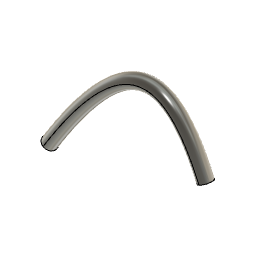
Final assembly_1001 (Autodesk Fusion 360 archive; units mm, degrees)
design "Blow Pipe_1001"
Autodesk Fusion 360 part; units mm, degrees
sketch "Sketch1" plane through (0, 0, 0) normal (0, 1, 0) x (1, 0, 0)
  spline S0 degree 5 poles (0, 0) (-0.9955, -2.3111) (-3.0243, -6.6799) (-6.1809, -12.4734) (-10.6201, -18.6535) (-16.5766, -23.6475) (-22.9681, -25.7259) (-29.8145, -24.7556) (-37.1022, -20.8271) (-44.7943, -14.1881) (-52.8502, -5.111) (-59.5578, 3.9127) (-64.7263, 11.6033) (-68.2321, 17.1339) (-70, 20) knots 0 0 0 0 0 0 0.1 0.2 0.3 0.4 0.5 0.6 0.7 0.8 0.9 1 1 1 1 1 1
  point P0 (-25, -25)
  constraint coincident S0.start origin
pipe "Pipe1" add diameter 6 wall 1 path "Sketch1" along S0

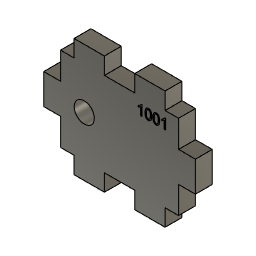
design "Housing block blowtube side version 2"
Autodesk Fusion 360 part; units mm, degrees
sketch "Sketch1" plane through (0, 0, 0) normal (0, 1, 0) x (1, 0, 0)
  line L0 (9, -55) -> (9, -50)
  line L1 (9, -50) -> (5, -50)
  line L2 (36, -55) -> (36, -50)
  line L3 (36, -50) -> (40, -50)
  line L4 (9, -55) -> (18, -55)
  line L5 (18, -55) -> (18, -50)
  line L6 (18, -50) -> (27, -50)
  line L7 (27, -50) -> (27, -55)
  line L8 (9, -55) -> (18, -55)
  line L9 (27, -55) -> (36, -55)
  line L10 (4, -42) -> (0, -42)
  line L11 (41, -42) -> (45, -42)
  line L12 (0, -42) -> (0, -37.5)
  line L13 (45, -42) -> (45, -37.5)
  line L14 (0, -37.5) -> (45, -37.5) construction
  line L15 (4, -42) -> (5, -42)
  line L16 (5, -42) -> (5, -50)
  line L17 (41, -42) -> (40, -42)
  line L18 (40, -42) -> (40, -50)
  line L19 (9, -20) -> (18, -20)
  line L20 (5, -33) -> (5, -25)
  line L21 (41, -33) -> (40, -33)
  line L22 (9, -25) -> (5, -25)
  line L23 (36, -20) -> (36, -25)
  line L24 (40, -33) -> (40, -25)
  line L25 (27, -25) -> (27, -20)
  line L26 (4, -33) -> (5, -33)
  line L27 (18, -25) -> (27, -25)
  line L28 (18, -20) -> (18, -25)
  line L29 (27, -20) -> (36, -20)
  line L30 (9, -20) -> (9, -25)
  line L31 (36, -25) -> (40, -25)
  line L32 (9, -20) -> (18, -20)
  line L33 (41, -33) -> (45, -33)
  line L34 (4, -33) -> (0, -33)
  line L35 (45, -33) -> (45, -37.5)
  line L36 (0, -33) -> (0, -37.5)
  dimension "d3" = 4.5
  dimension "d4" = 4.5
  constraint horizontal L8
  constraint vertical L0
  constraint horizontal L1
  constraint vertical L2
  constraint horizontal L3
  constraint perpendicular L4 L5
  constraint perpendicular L5 L6
  constraint coincident L7.end L8
  constraint perpendicular L7 L8
  constraint collinear L8 L9
  constraint perpendicular L10 L12
  constraint perpendicular L11 L13
  constraint perpendicular L13 L14
  constraint perpendicular L1 L16
  constraint perpendicular L3 L18
  constraint symmetric L0.start L14 L19.start
  constraint symmetric L0.end L14 L22.start
  constraint symmetric L2.start L14 L23.start
  constraint symmetric L2.end L14 L23.end
  constraint symmetric L4.end L14 L19.end
  constraint symmetric L5.end L14 L27.start
  constraint symmetric L6.end L14 L25.start
  constraint symmetric L7.end L14 L25.end
  constraint symmetric L10.start L14 L26.start
  constraint symmetric L10.end L14 L34.end
  constraint symmetric L11.start L14 L21.start
  constraint symmetric L11.end L14 L33.end
  constraint symmetric L12.end L14 L36.end
  constraint symmetric L13.end L14 L35.end
  constraint symmetric L14 L15.end L20.start
  constraint symmetric L14 L1.end L20.end
  constraint symmetric L14 L17.end L21.end
  constraint symmetric L14 L3.end L24.end
  measures "d3" distance of L10.end L12.end
  measures "d4" distance of L11.end L13.end
extrude "Extrude1" add sketch "Sketch1" along normal blind 5
sketch "Sketch2" plane through (0, 0, 0) normal (0, -1, 0) x (1, 0, 0)
  line L0 (0, 33) -> (5, 33)
  line L1 (5, 33) -> (5, 25)
  line L2 (5, 25) -> (9, 25)
  line L3 (9, 25) -> (9, 20)
  line L4 (9, 20) -> (18, 20)
  line L5 (18, 20) -> (18, 25)
  line L6 (18, 25) -> (27, 25)
  line L7 (27, 25) -> (27, 20)
  line L8 (27, 20) -> (36, 20)
  line L9 (36, 20) -> (36, 25)
  line L10 (36, 25) -> (40, 25)
  line L11 (40, 25) -> (40, 33)
  line L12 (40, 33) -> (45, 33)
  line L13 (45, 33) -> (45, 42)
  line L14 (45, 42) -> (40, 42)
  line L15 (40, 42) -> (40, 50)
  line L16 (40, 50) -> (36, 50)
  line L17 (36, 50) -> (36, 55)
  line L18 (36, 55) -> (27, 55)
  line L19 (27, 55) -> (27, 50)
  line L20 (27, 50) -> (18, 50)
  line L21 (18, 50) -> (18, 55)
  line L22 (18, 55) -> (9, 55)
  line L23 (9, 55) -> (9, 50)
  line L24 (9, 50) -> (5, 50)
  line L25 (5, 50) -> (5, 42)
  line L26 (5, 42) -> (0, 42)
  line L27 (0, 42) -> (0, 33)
  circle A0 centre (12.027, 37.5) radius 3
  dimension "d7" = 6
  measures "d7" diameter of A0
extrude "Extrude2" cut sketch "Sketch2" against normal blind 5 contours A0
sketch "Sketch3" plane through (0, 0, 0) normal (0, -1, 0) x (1, 0, 0)
  circle A0 centre (12.027, 37.5) radius 3
  line L0 (0, 33) -> (5, 33)
  line L1 (5, 33) -> (5, 25)
  line L2 (5, 25) -> (9, 25)
  line L3 (9, 25) -> (9, 20)
  line L4 (9, 20) -> (18, 20)
  line L5 (18, 20) -> (18, 25)
  line L6 (18, 25) -> (27, 25)
  line L7 (27, 25) -> (27, 20)
  line L8 (27, 20) -> (36, 20)
  line L9 (36, 20) -> (36, 25)
  line L10 (36, 25) -> (40, 25)
  line L11 (40, 25) -> (40, 33)
  line L12 (40, 33) -> (45, 33)
  line L13 (45, 33) -> (45, 42)
  line L14 (45, 42) -> (40, 42)
  line L15 (40, 42) -> (40, 50)
  line L16 (40, 50) -> (36, 50)
  line L17 (36, 50) -> (36, 55)
  line L18 (36, 55) -> (27, 55)
  line L19 (27, 55) -> (27, 50)
  line L20 (27, 50) -> (18, 50)
  line L21 (18, 50) -> (18, 55)
  line L22 (18, 55) -> (9, 55)
  line L23 (9, 55) -> (9, 50)
  line L24 (9, 50) -> (5, 50)
  line L25 (5, 50) -> (5, 42)
  line L26 (5, 42) -> (0, 42)
  line L27 (0, 42) -> (0, 33)
  line L28 (27.9971, 44.0065) -> (37, 44) construction
  line L29 (37, 44) -> (37.0029, 47.9935) construction
  line L30 (37.0029, 47.9935) -> (28, 48) construction
  line L31 (28, 48) -> (27.9971, 44.0065) construction
  dimension "d10" = 3
  text T0 "1001" font "Arial" height 3 align left top in box 9.0029 x 3.9935 at (27.9971, 44.0065) x (1, -0.000717) y (0.000717, 1) spacing 1 kerned
emboss "Emboss1" depth -0.1 profiles "Sketch3" section 1 text T0 onto face at (31.3333, 0, 36)

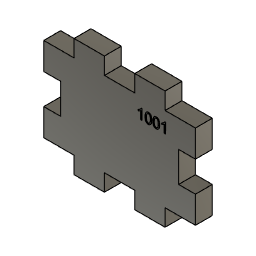
design "Housing block top and bottom version 2"
Autodesk Fusion 360 part; units mm, degrees
sketch "Sketch1" plane through (0, 0, 0) normal (0, 1, 0) x (1, 0, 0)
  line L0 (45, -22) -> (45, -30)
  line L1 (0, -30) -> (9, -30)
  line L2 (9, -30) -> (9, -35)
  line L3 (9, -35) -> (18, -35)
  line L4 (18, -35) -> (18, -30)
  line L5 (18, -30) -> (27, -30)
  line L6 (27, -30) -> (27, -35)
  line L7 (36, -35) -> (27, -35)
  line L8 (18, -35) -> (9, -35)
  line L9 (36, -35) -> (36, -30)
  line L10 (36, -30) -> (45, -30)
  line L11 (0, -30) -> (0, -22)
  line L12 (5, -22) -> (5, -17.5)
  line L13 (45, -30) -> (45, -22)
  line L14 (40, -22) -> (40, -17.5)
  line L15 (40, -22) -> (45, -22)
  line L16 (5, -17.5) -> (40, -17.5) construction
  line L17 (18, 0) -> (9, 0)
  line L18 (27, -5) -> (27, 0)
  line L19 (36, -5) -> (45, -5)
  line L20 (36, 0) -> (27, 0)
  line L21 (18, 0) -> (18, -5)
  line L22 (9, 0) -> (18, 0)
  line L23 (40, -13) -> (45, -13)
  line L24 (0, -5) -> (0, -13)
  line L25 (18, -5) -> (27, -5)
  line L26 (0, -5) -> (9, -5)
  line L27 (40, -13) -> (40, -17.5)
  line L28 (36, 0) -> (36, -5)
  line L29 (5, -13) -> (5, -17.5)
  line L30 (9, -5) -> (9, 0)
  line L31 (45, -5) -> (45, -13)
  line L32 (0, -22) -> (5, -22)
  line L33 (5, -13) -> (0, -13)
  dimension "d3" = 4.5
  dimension "d4" = 4.5
  constraint vertical L0
  constraint horizontal L7
  constraint coincident L2.end L7
  constraint perpendicular L2 L7
  constraint coincident L3.end L7
  constraint perpendicular L3 L4
  constraint perpendicular L4 L5
  constraint perpendicular L6 L7
  constraint collinear L7 L8
  constraint perpendicular L7 L9
  constraint perpendicular L0 L10
  constraint perpendicular L1 L12
  constraint perpendicular L10 L14
  constraint perpendicular L13 L15
  constraint perpendicular L12 L16
  constraint symmetric L1.start L16 L24.start
  constraint symmetric L1.end L16 L26.end
  constraint symmetric L2.end L16 L17.end
  constraint symmetric L3.end L16 L17.start
  constraint symmetric L4.end L16 L21.end
  constraint symmetric L5.end L16 L18.start
  constraint symmetric L6.end L16 L18.end
  constraint symmetric L7.start L16 L20.start
  constraint symmetric L9.end L16 L19.start
  constraint symmetric L0.end L16 L19.end
  constraint symmetric L11.end L16 L24.end
  constraint symmetric L12.start L16 L29.start
  constraint symmetric L12.end L16 L29.end
  constraint symmetric L0.start L16 L23.end
  constraint symmetric L14.start L16 L23.start
  constraint symmetric L14.end L16 L27.end
  constraint perpendicular L11 L32
  measures "d3" distance of L12.start L12.end
  measures "d4" distance of L14.start L14.end
extrude "Extrude1" add sketch "Sketch1" along normal blind 5
sketch "Sketch2" plane through (0, 0, 0) normal (0, -1, 0) x (1, 0, 0)
  line L0 (9, 30) -> (0, 30)
  line L1 (0, 30) -> (0, 22)
  line L2 (0, 22) -> (5, 22)
  line L3 (5, 22) -> (5, 13)
  line L4 (5, 13) -> (0, 13)
  line L5 (0, 13) -> (0, 5)
  line L6 (0, 5) -> (9, 5)
  line L7 (9, 5) -> (9, 0)
  line L8 (9, 0) -> (18, 0)
  line L9 (18, 0) -> (18, 5)
  line L10 (18, 5) -> (27, 5)
  line L11 (27, 5) -> (27, 0)
  line L12 (27, 0) -> (36, 0)
  line L13 (36, 0) -> (36, 5)
  line L14 (36, 5) -> (45, 5)
  line L15 (45, 5) -> (45, 13)
  line L16 (45, 13) -> (40, 13)
  line L17 (40, 13) -> (40, 22)
  line L18 (40, 22) -> (45, 22)
  line L19 (45, 22) -> (45, 30)
  line L20 (45, 30) -> (36, 30)
  line L21 (36, 30) -> (36, 35)
  line L22 (36, 35) -> (27, 35)
  line L23 (27, 35) -> (27, 30)
  line L24 (27, 30) -> (18, 30)
  line L25 (18, 30) -> (18, 35)
  line L26 (18, 35) -> (9, 35)
  line L27 (9, 35) -> (9, 30)
  line L28 (27.994, 23.0136) -> (37, 23) construction
  line L29 (37, 23) -> (37.006, 26.9864) construction
  line L30 (37.006, 26.9864) -> (28, 27) construction
  line L31 (28, 27) -> (27.994, 23.0136) construction
  dimension "d7" = 3
  text T0 "1001" font "Arial" height 3 align left top in box 9.006 x 3.9864 at (27.994, 23.0136) x (0.999999, -0.001514) y (0.001514, 0.999999) spacing 1 kerned
emboss "Emboss1" depth -0.1 profiles "Sketch2" section 1 text T0 onto face at (13.6667, 0, 17.5)

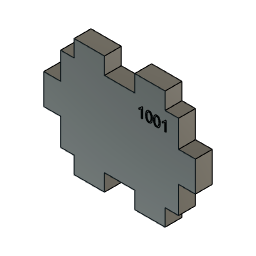
design "Housing block other side version 2"
Autodesk Fusion 360 part; units mm, degrees
sketch "Sketch1" plane through (0, 0, 0) normal (0, 1, 0) x (1, 0, 0)
  line L0 (9, -55) -> (9, -50)
  line L1 (9, -50) -> (5, -50)
  line L2 (36, -55) -> (36, -50)
  line L3 (36, -50) -> (40, -50)
  line L4 (9, -55) -> (18, -55)
  line L5 (18, -55) -> (18, -50)
  line L6 (18, -50) -> (27, -50)
  line L7 (27, -50) -> (27, -55)
  line L8 (9, -55) -> (18, -55)
  line L9 (27, -55) -> (36, -55)
  line L10 (4, -42) -> (0, -42)
  line L11 (41, -42) -> (45, -42)
  line L12 (0, -42) -> (0, -37.5)
  line L13 (45, -42) -> (45, -37.5)
  line L14 (0, -37.5) -> (45, -37.5) construction
  line L15 (4, -42) -> (5, -42)
  line L16 (5, -42) -> (5, -50)
  line L17 (41, -42) -> (40, -42)
  line L18 (40, -42) -> (40, -50)
  line L19 (9, -20) -> (18, -20)
  line L20 (5, -33) -> (5, -25)
  line L21 (41, -33) -> (40, -33)
  line L22 (9, -25) -> (5, -25)
  line L23 (36, -20) -> (36, -25)
  line L24 (40, -33) -> (40, -25)
  line L25 (27, -25) -> (27, -20)
  line L26 (4, -33) -> (5, -33)
  line L27 (18, -25) -> (27, -25)
  line L28 (18, -20) -> (18, -25)
  line L29 (27, -20) -> (36, -20)
  line L30 (9, -20) -> (9, -25)
  line L31 (36, -25) -> (40, -25)
  line L32 (9, -20) -> (18, -20)
  line L33 (41, -33) -> (45, -33)
  line L34 (4, -33) -> (0, -33)
  line L35 (45, -33) -> (45, -37.5)
  line L36 (0, -33) -> (0, -37.5)
  dimension "d3" = 4.5
  dimension "d4" = 4.5
  constraint horizontal L8
  constraint vertical L0
  constraint horizontal L1
  constraint vertical L2
  constraint horizontal L3
  constraint perpendicular L4 L5
  constraint perpendicular L5 L6
  constraint coincident L7.end L8
  constraint perpendicular L7 L8
  constraint collinear L8 L9
  constraint perpendicular L10 L12
  constraint perpendicular L11 L13
  constraint perpendicular L13 L14
  constraint perpendicular L1 L16
  constraint perpendicular L3 L18
  constraint symmetric L0.start L14 L19.start
  constraint symmetric L0.end L14 L22.start
  constraint symmetric L2.start L14 L23.start
  constraint symmetric L2.end L14 L23.end
  constraint symmetric L4.end L14 L19.end
  constraint symmetric L5.end L14 L27.start
  constraint symmetric L6.end L14 L25.start
  constraint symmetric L7.end L14 L25.end
  constraint symmetric L10.start L14 L26.start
  constraint symmetric L10.end L14 L34.end
  constraint symmetric L11.start L14 L21.start
  constraint symmetric L11.end L14 L33.end
  constraint symmetric L12.end L14 L36.end
  constraint symmetric L13.end L14 L35.end
  constraint symmetric L14 L15.end L20.start
  constraint symmetric L14 L1.end L20.end
  constraint symmetric L14 L17.end L21.end
  constraint symmetric L14 L3.end L24.end
  measures "d3" distance of L10.end L12.end
  measures "d4" distance of L11.end L13.end
extrude "Extrude1" add sketch "Sketch1" along normal blind 5
sketch "Sketch2" plane through (0, 0, 0) normal (0, -1, 0) x (1, 0, 0)
  line L0 (0, 33) -> (5, 33)
  line L1 (5, 33) -> (5, 25)
  line L2 (5, 25) -> (9, 25)
  line L3 (9, 25) -> (9, 20)
  line L4 (9, 20) -> (18, 20)
  line L5 (18, 20) -> (18, 25)
  line L6 (18, 25) -> (27, 25)
  line L7 (27, 25) -> (27, 20)
  line L8 (27, 20) -> (36, 20)
  line L9 (36, 20) -> (36, 25)
  line L10 (36, 25) -> (40, 25)
  line L11 (40, 25) -> (40, 33)
  line L12 (40, 33) -> (45, 33)
  line L13 (45, 33) -> (45, 42)
  line L14 (45, 42) -> (40, 42)
  line L15 (40, 42) -> (40, 50)
  line L16 (40, 50) -> (36, 50)
  line L17 (36, 50) -> (36, 55)
  line L18 (36, 55) -> (27, 55)
  line L19 (27, 55) -> (27, 50)
  line L20 (27, 50) -> (18, 50)
  line L21 (18, 50) -> (18, 55)
  line L22 (18, 55) -> (9, 55)
  line L23 (9, 55) -> (9, 50)
  line L24 (9, 50) -> (5, 50)
  line L25 (5, 50) -> (5, 42)
  line L26 (5, 42) -> (0, 42)
  line L27 (0, 42) -> (0, 33)
sketch "Sketch3" plane through (0, 0, 0) normal (0, -1, 0) x (1, 0, 0)
  line L0 (28.1867, 44.4859) -> (37.0015, 44.4949) construction
  line L1 (37.0015, 44.4949) -> (36.9985, 47.5051) construction
  line L2 (36.9985, 47.5051) -> (28.1836, 47.4961) construction
  line L3 (28.1836, 47.4961) -> (28.1867, 44.4859) construction
  dimension "d8" = 3
  text T0 "1001" font "Arial" height 3 align left top in box 8.8149 x 3.0103 at (28.1867, 44.4859) x (0.999999, 0.00102) y (-0.00102, 0.999999) spacing 1 kerned
emboss "Emboss1" depth -0.1 profiles "Sketch3" section 1 text T0 onto face at (13.6667, 0, 36)

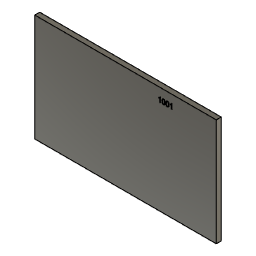
design "Base Plate"
Autodesk Fusion 360 part; units mm, degrees
sketch "Sketch1" plane through (0, 0, 0) normal (0, 1, 0) x (1, 0, 0)
  line L0 (-40, -25) -> (70, -25)
  line L1 (70, -25) -> (70, -90)
  line L2 (70, -90) -> (-40, -90)
  line L3 (-40, -90) -> (-40, -25)
  dimension "d1" = 110
  dimension "d2" = 65
  constraint horizontal L0
  constraint vertical L1
  constraint horizontal L2
  constraint vertical L3
  measures "d1" distance of L0.start L0.end
  measures "d2" distance of L0.start L2.end
extrude "Extrude1" add sketch "Sketch1" along normal blind 3
sketch "Sketch2" plane through (0, 0, 0) normal (0, -1, 0) x (1, 0, 0)
  line L0 (70, 90) -> (-40, 90)
  line L1 (-40, 90) -> (-40, 25)
  line L2 (-40, 25) -> (70, 25)
  line L3 (70, 25) -> (70, 90)
  line L4 (35, 75.5912) -> (62.1454, 75.5912) construction
  line L5 (62.1454, 75.5912) -> (62.1454, 85) construction
  line L6 (62.1454, 85) -> (35, 85) construction
  line L7 (35, 85) -> (35, 75.5912) construction
  dimension "d5" = 3
  text T0 "1001" font "Arial" height 3 align left top in box 27.1454 x 9.4088 at (35, 75.5912) x (1, 0) y (0, 1) spacing 1 kerned
emboss "Emboss1" depth -0.5 profiles "Sketch2" section 1 text T0 onto face at (-3.3333, 0, 46.6667)

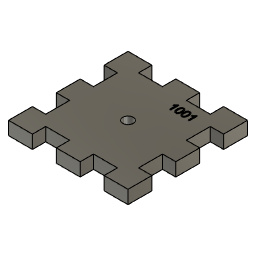
design "Housing_back"
Autodesk Fusion 360 part; units mm, degrees
sketch "Sketch1" plane through (0, 0, 0) normal (0, 0, 1) x (1, 0, 0)
  line L0 (0, 0) -> (9, 0)
  line L1 (9, 0) -> (9, -5)
  line L2 (9, -5) -> (18, -5)
  line L3 (18, -5) -> (18, 0)
  line L4 (18, 0) -> (27, 0)
  line L5 (27, 0) -> (27, -5)
  line L6 (27, -5) -> (36, -5)
  line L7 (36, -5) -> (36, 0)
  line L8 (36, 0) -> (45, 0)
  line L9 (45, 0) -> (45, -9)
  line L10 (45, -9) -> (40, -9)
  line L11 (40, -9) -> (40, -18)
  line L12 (40, -18) -> (45, -18)
  line L13 (45, -18) -> (45, -27)
  line L14 (45, -27) -> (40, -27)
  line L15 (40, -27) -> (40, -36)
  line L16 (40, -36) -> (45, -36)
  line L17 (45, -36) -> (45, -45)
  line L18 (50, 0) -> (50, -22.5) construction
  line L19 (50, -22.5) -> (-20, -22.5) construction
  line L20 (0, -45) -> (9, -45)
  line L21 (9, -45) -> (9, -40)
  line L22 (9, -40) -> (18, -40)
  line L23 (18, -40) -> (18, -45)
  line L24 (18, -45) -> (27, -45)
  line L25 (27, -45) -> (27, -40)
  line L26 (27, -40) -> (36, -40)
  line L27 (36, -40) -> (36, -45)
  line L28 (36, -45) -> (45, -45)
  line L29 (50, 0) -> (27.5, 0) construction
  line L30 (45, 10) -> (22.5, 10) construction
  line L31 (22.5, 10) -> (22.5, -55) construction
  line L32 (0, 0) -> (0, -9)
  line L33 (0, -9) -> (5, -9)
  line L34 (5, -9) -> (5, -18)
  line L35 (5, -18) -> (0, -18)
  line L36 (0, -18) -> (0, -27)
  line L37 (0, -27) -> (5, -27)
  line L38 (5, -27) -> (5, -36)
  line L39 (5, -36) -> (0, -36)
  line L40 (0, -36) -> (0, -45)
  dimension "d1" = 9
  dimension "d2" = 5
  dimension "d3" = 9
  dimension "d4" = 5
  dimension "d5" = 9
  dimension "d6" = 5
  dimension "d7" = 9
  dimension "d8" = 5
  dimension "d9" = 9
  dimension "d10" = 9
  dimension "d11" = 5
  dimension "d12" = 9
  dimension "d13" = 9
  dimension "d14" = 5
  dimension "d15" = 9
  dimension "d16" = 9
  dimension "d17" = 22.5
  dimension "d18" = 22.5
  dimension "d19" = 22.5
  constraint coincident L0.start L32.start
  constraint horizontal L0
  constraint perpendicular L0 L1
  constraint perpendicular L1 L2
  constraint perpendicular L2 L3
  constraint perpendicular L3 L4
  constraint perpendicular L4 L5
  constraint perpendicular L5 L6
  constraint perpendicular L6 L7
  constraint perpendicular L7 L8
  constraint perpendicular L8 L9
  constraint perpendicular L9 L10
  constraint perpendicular L10 L11
  constraint perpendicular L11 L12
  constraint perpendicular L12 L13
  constraint perpendicular L13 L14
  constraint perpendicular L14 L15
  constraint perpendicular L15 L16
  constraint perpendicular L16 L17
  constraint vertical L18
  constraint perpendicular L18 L19
  constraint symmetric L0.start L19 L20.start
  constraint symmetric L0.end L19 L20.end
  constraint symmetric L1.end L19 L21.end
  constraint symmetric L2.end L19 L22.end
  constraint symmetric L3.end L19 L23.end
  constraint symmetric L4.end L19 L24.end
  constraint symmetric L5.end L19 L25.end
  constraint symmetric L6.end L19 L26.end
  constraint symmetric L7.end L19 L27.end
  constraint symmetric L8.end L19 L17.end
  constraint perpendicular L9 L29
  constraint perpendicular L9 L30
  constraint perpendicular L24 L31
  constraint symmetric L8.end L31 L0.start
  constraint symmetric L9.end L31 L32.end
  constraint symmetric L10.end L31 L33.end
  constraint symmetric L11.end L31 L34.end
  constraint symmetric L12.end L31 L35.end
  constraint symmetric L13.end L31 L36.end
  constraint symmetric L14.end L31 L37.end
  constraint symmetric L15.end L31 L38.end
  constraint symmetric L16.end L31 L39.end
  constraint symmetric L17.end L31 L20.start
  measures "d1" distance of L0.start L0.end
  measures "d2" distance of L0.end L1.end
  measures "d3" distance of L1.end L2.end
  measures "d4" distance of L2.end L3.end
  measures "d5" distance of L3.end L4.end
  measures "d6" distance of L4.end L5.end
  measures "d7" distance of L5.end L6.end
  measures "d8" distance of L6.end L7.end
  measures "d9" distance of L7.end L8.end
  measures "d10" distance of L8.end L9.end
  measures "d11" distance of L9.end L10.end
  measures "d12" distance of L10.end L11.end
  measures "d13" distance of L12.end L13.end
  measures "d14" distance of L13.end L14.end
  measures "d15" distance of L14.end L15.end
  measures "d16" distance of L16.end L17.end
  measures "d17" distance of L18.start L18.end
  measures "d18" distance of L18.start L29.end
  measures "d19" distance of L30.start L30.end
extrude "Extrude1" add sketch "Sketch1" along normal blind 5
sketch "Sketch2" plane through (0, 0, 5) normal (0, 0, 1) x (-1, 0, 0)
  line L0 (0, 0) -> (0, 9)
  line L1 (0, 9) -> (-5, 9)
  line L2 (-5, 9) -> (-5, 18)
  line L3 (-5, 18) -> (0, 18)
  line L4 (0, 18) -> (0, 27)
  line L5 (0, 27) -> (-5, 27)
  line L6 (-5, 27) -> (-5, 36)
  line L7 (-5, 36) -> (0, 36)
  line L8 (0, 36) -> (0, 45)
  line L9 (0, 45) -> (-9, 45)
  line L10 (-9, 45) -> (-9, 40)
  line L11 (-9, 40) -> (-18, 40)
  line L12 (-18, 40) -> (-18, 45)
  line L13 (-18, 45) -> (-27, 45)
  line L14 (-27, 45) -> (-27, 40)
  line L15 (-27, 40) -> (-36, 40)
  line L16 (-36, 40) -> (-36, 45)
  line L17 (-36, 45) -> (-45, 45)
  line L18 (-45, 45) -> (-45, 36)
  line L19 (-45, 36) -> (-40, 36)
  line L20 (-40, 36) -> (-40, 27)
  line L21 (-40, 27) -> (-45, 27)
  line L22 (-45, 27) -> (-45, 18)
  line L23 (-45, 18) -> (-40, 18)
  line L24 (-40, 18) -> (-40, 9)
  line L25 (-40, 9) -> (-45, 9)
  line L26 (-45, 9) -> (-45, 0)
  line L27 (-45, 0) -> (-36, 0)
  line L28 (-36, 0) -> (-36, 5)
  line L29 (-36, 5) -> (-27, 5)
  line L30 (-27, 5) -> (-27, 0)
  line L31 (-27, 0) -> (-18, 0)
  line L32 (-18, 0) -> (-18, 5)
  line L33 (-18, 5) -> (-9, 5)
  line L34 (-9, 5) -> (-9, 0)
  line L35 (-9, 0) -> (0, 0)
  circle A0 centre (-22.5, 22.5) radius 2
  dimension "d22" = 4
  measures "d22" diameter of A0
extrude "Extrude2" cut sketch "Sketch2" against normal blind 5 contours A0
sketch "Sketch3" plane through (0, 0, 5) normal (0, 0, 1) x (-1, 0, 0)
  circle A0 centre (-22.5, 22.5) radius 2
  line L0 (0, 0) -> (0, 9)
  line L1 (0, 9) -> (-5, 9)
  line L2 (-5, 9) -> (-5, 18)
  line L3 (-5, 18) -> (0, 18)
  line L4 (0, 18) -> (0, 27)
  line L5 (0, 27) -> (-5, 27)
  line L6 (-5, 27) -> (-5, 36)
  line L7 (-5, 36) -> (0, 36)
  line L8 (0, 36) -> (0, 45)
  line L9 (0, 45) -> (-9, 45)
  line L10 (-9, 45) -> (-9, 40)
  line L11 (-9, 40) -> (-18, 40)
  line L12 (-18, 40) -> (-18, 45)
  line L13 (-18, 45) -> (-27, 45)
  line L14 (-27, 45) -> (-27, 40)
  line L15 (-27, 40) -> (-36, 40)
  line L16 (-36, 40) -> (-36, 45)
  line L17 (-36, 45) -> (-45, 45)
  line L18 (-45, 45) -> (-45, 36)
  line L19 (-45, 36) -> (-40, 36)
  line L20 (-40, 36) -> (-40, 27)
  line L21 (-40, 27) -> (-45, 27)
  line L22 (-45, 27) -> (-45, 18)
  line L23 (-45, 18) -> (-40, 18)
  line L24 (-40, 18) -> (-40, 9)
  line L25 (-40, 9) -> (-45, 9)
  line L26 (-45, 9) -> (-45, 0)
  line L27 (-45, 0) -> (-36, 0)
  line L28 (-36, 0) -> (-36, 5)
  line L29 (-36, 5) -> (-27, 5)
  line L30 (-27, 5) -> (-27, 0)
  line L31 (-27, 0) -> (-18, 0)
  line L32 (-18, 0) -> (-18, 5)
  line L33 (-18, 5) -> (-9, 5)
  line L34 (-9, 5) -> (-9, 0)
  line L35 (-9, 0) -> (0, 0)
  line L36 (-25.9904, 10.9709) -> (-35, 11) construction
  line L37 (-35, 11) -> (-35.0096, 8.0291) construction
  line L38 (-35.0096, 8.0291) -> (-26, 8) construction
  line L39 (-26, 8) -> (-25.9904, 10.9709) construction
  dimension "d25" = 3
  text T0 "1001\n" font "Arial" height 3 align left top in box 9.0096 x 2.9709 at (-25.9904, 10.9709) x (-0.999995, 0.003232) y (-0.003232, -0.999995) spacing 1 kerned
emboss "Emboss1" depth -0.1 profiles "Sketch3" section 1 text T0 onto face at (30.322, -30.2868, 5)

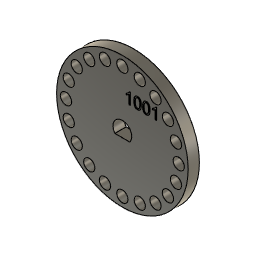
design "Slotted disk final version"
Autodesk Fusion 360 part; units mm, degrees
sketch "Sketch1" plane through (0, 0, 0) normal (0, 1, 0) x (1, 0, 0)
  circle A0 centre (0, 0) radius 17.5
  circle A1 centre (0, -15) radius 1.5
  circle A2 centre (4.6353, -14.2658) radius 1.5
  circle A3 centre (8.8168, -12.1353) radius 1.5
  circle A4 centre (12.1353, -8.8168) radius 1.5
  circle A5 centre (14.2658, -4.6353) radius 1.5
  circle A6 centre (15, 0) radius 1.5
  circle A7 centre (14.2658, 4.6353) radius 1.5
  circle A8 centre (12.1353, 8.8168) radius 1.5
  circle A9 centre (8.8168, 12.1353) radius 1.5
  circle A10 centre (4.6353, 14.2658) radius 1.5
  circle A11 centre (0, 15) radius 1.5
  circle A12 centre (-4.6353, 14.2658) radius 1.5
  circle A13 centre (-8.8168, 12.1353) radius 1.5
  circle A14 centre (-12.1353, 8.8168) radius 1.5
  circle A15 centre (-14.2658, 4.6353) radius 1.5
  circle A16 centre (-15, 0) radius 1.5
  circle A17 centre (-14.2658, -4.6353) radius 1.5
  circle A18 centre (-12.1353, -8.8168) radius 1.5
  circle A19 centre (-8.8168, -12.1353) radius 1.5
  circle A20 centre (-4.6353, -14.2658) radius 1.5
  line L0 (0, 0) -> (0, 1.5) construction
  line L1 (0, 1.5) -> (2, 1.5)
  line L2 (-2, 1.5) -> (0, 1.5)
  arc A21 (-2, 1.5) -> (2, 1.5) centre (0, 0) ccw
  dimension "d1" = 35
  dimension "d2" = 15
  dimension "d3" = 3
  dimension "d5" = 360
  dimension "d6" = 5
  dimension "d7" = 1.5
  constraint coincident A0.centre L0.start
  constraint perpendicular L0 L1
  constraint perpendicular L0 L2
  measures "d1" diameter of A0
  measures "d2" distance of A0.centre A1.centre
  measures "d3" diameter of A1
  measures "d6" diameter of A21
  measures "d7" distance of A0.centre L0.end
extrude "Extrude1" add sketch "Sketch1" along normal blind 3
sketch "Sketch2" plane through (0, 0, 0) normal (0, 1, 0) x (1, 0, 0)
  line L0 (1, -7) -> (9, -7) construction
  line L1 (9, -7) -> (9, -10) construction
  line L2 (9, -10) -> (1, -10) construction
  line L3 (1, -10) -> (1, -7) construction
  dimension "d10" = 3
  text T0 "1001" font "Arial" height 3 align left top in box 8 x 3 at (1, -7) x (1, 0) y (0, -1) spacing 1 kerned
emboss "Emboss1" depth -0.1 profiles "Sketch2" section 1 text T0 onto face at (-6.9502, 0, -6.8341)

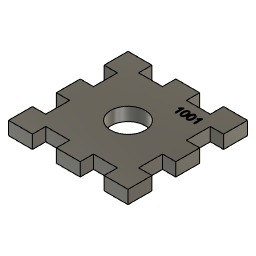
design "Housing_front"
Autodesk Fusion 360 part; units mm, degrees
sketch "Sketch1" plane through (0, 0, 0) normal (0, 0, 1) x (1, 0, 0)
  line L0 (0, 0) -> (9, 0)
  line L1 (9, 0) -> (9, -5)
  line L2 (9, -5) -> (18, -5)
  line L3 (18, -5) -> (18, 0)
  line L4 (18, 0) -> (27, 0)
  line L5 (27, 0) -> (27, -5)
  line L6 (27, -5) -> (36, -5)
  line L7 (36, -5) -> (36, 0)
  line L8 (36, 0) -> (45, 0)
  line L9 (45, 0) -> (45, -9)
  line L10 (45, -9) -> (40, -9)
  line L11 (40, -9) -> (40, -18)
  line L12 (40, -18) -> (45, -18)
  line L13 (45, -18) -> (45, -27)
  line L14 (45, -27) -> (40, -27)
  line L15 (40, -27) -> (40, -36)
  line L16 (40, -36) -> (45, -36)
  line L17 (45, -36) -> (45, -45)
  line L18 (50, 0) -> (50, -22.5) construction
  line L19 (50, -22.5) -> (-20, -22.5) construction
  line L20 (0, -45) -> (9, -45)
  line L21 (9, -45) -> (9, -40)
  line L22 (9, -40) -> (18, -40)
  line L23 (18, -40) -> (18, -45)
  line L24 (18, -45) -> (27, -45)
  line L25 (27, -45) -> (27, -40)
  line L26 (27, -40) -> (36, -40)
  line L27 (36, -40) -> (36, -45)
  line L28 (36, -45) -> (45, -45)
  line L29 (50, 0) -> (27.5, 0) construction
  line L30 (45, 10) -> (22.5, 10) construction
  line L31 (22.5, 10) -> (22.5, -55) construction
  line L32 (0, 0) -> (0, -9)
  line L33 (0, -9) -> (5, -9)
  line L34 (5, -9) -> (5, -18)
  line L35 (5, -18) -> (0, -18)
  line L36 (0, -18) -> (0, -27)
  line L37 (0, -27) -> (5, -27)
  line L38 (5, -27) -> (5, -36)
  line L39 (5, -36) -> (0, -36)
  line L40 (0, -36) -> (0, -45)
  dimension "d1" = 9
  dimension "d2" = 5
  dimension "d3" = 9
  dimension "d4" = 5
  dimension "d5" = 9
  dimension "d6" = 5
  dimension "d7" = 9
  dimension "d8" = 5
  dimension "d9" = 9
  dimension "d10" = 9
  dimension "d11" = 5
  dimension "d12" = 9
  dimension "d13" = 9
  dimension "d14" = 5
  dimension "d15" = 9
  dimension "d16" = 9
  dimension "d17" = 22.5
  dimension "d18" = 22.5
  dimension "d19" = 22.5
  constraint coincident L0.start L32.start
  constraint horizontal L0
  constraint perpendicular L0 L1
  constraint perpendicular L1 L2
  constraint perpendicular L2 L3
  constraint perpendicular L3 L4
  constraint perpendicular L4 L5
  constraint perpendicular L5 L6
  constraint perpendicular L6 L7
  constraint perpendicular L7 L8
  constraint perpendicular L8 L9
  constraint perpendicular L9 L10
  constraint perpendicular L10 L11
  constraint perpendicular L11 L12
  constraint perpendicular L12 L13
  constraint perpendicular L13 L14
  constraint perpendicular L14 L15
  constraint perpendicular L15 L16
  constraint perpendicular L16 L17
  constraint vertical L18
  constraint perpendicular L18 L19
  constraint symmetric L0.start L19 L20.start
  constraint symmetric L0.end L19 L20.end
  constraint symmetric L1.end L19 L21.end
  constraint symmetric L2.end L19 L22.end
  constraint symmetric L3.end L19 L23.end
  constraint symmetric L4.end L19 L24.end
  constraint symmetric L5.end L19 L25.end
  constraint symmetric L6.end L19 L26.end
  constraint symmetric L7.end L19 L27.end
  constraint symmetric L8.end L19 L17.end
  constraint perpendicular L9 L29
  constraint perpendicular L9 L30
  constraint perpendicular L24 L31
  constraint symmetric L8.end L31 L0.start
  constraint symmetric L9.end L31 L32.end
  constraint symmetric L10.end L31 L33.end
  constraint symmetric L11.end L31 L34.end
  constraint symmetric L12.end L31 L35.end
  constraint symmetric L13.end L31 L36.end
  constraint symmetric L14.end L31 L37.end
  constraint symmetric L15.end L31 L38.end
  constraint symmetric L16.end L31 L39.end
  constraint symmetric L17.end L31 L20.start
  measures "d1" distance of L0.start L0.end
  measures "d2" distance of L0.end L1.end
  measures "d3" distance of L1.end L2.end
  measures "d4" distance of L2.end L3.end
  measures "d5" distance of L3.end L4.end
  measures "d6" distance of L4.end L5.end
  measures "d7" distance of L5.end L6.end
  measures "d8" distance of L6.end L7.end
  measures "d9" distance of L7.end L8.end
  measures "d10" distance of L8.end L9.end
  measures "d11" distance of L9.end L10.end
  measures "d12" distance of L10.end L11.end
  measures "d13" distance of L12.end L13.end
  measures "d14" distance of L13.end L14.end
  measures "d15" distance of L14.end L15.end
  measures "d16" distance of L16.end L17.end
  measures "d17" distance of L18.start L18.end
  measures "d18" distance of L18.start L29.end
  measures "d19" distance of L30.start L30.end
extrude "Extrude1" add sketch "Sketch1" along normal blind 5
sketch "Sketch2" plane through (0, 0, 5) normal (0, 0, 1) x (-1, 0, 0)
  line L0 (0, 0) -> (0, 9)
  line L1 (0, 9) -> (-5, 9)
  line L2 (-5, 9) -> (-5, 18)
  line L3 (-5, 18) -> (0, 18)
  line L4 (0, 18) -> (0, 27)
  line L5 (0, 27) -> (-5, 27)
  line L6 (-5, 27) -> (-5, 36)
  line L7 (-5, 36) -> (0, 36)
  line L8 (0, 36) -> (0, 45)
  line L9 (0, 45) -> (-9, 45)
  line L10 (-9, 45) -> (-9, 40)
  line L11 (-9, 40) -> (-18, 40)
  line L12 (-18, 40) -> (-18, 45)
  line L13 (-18, 45) -> (-27, 45)
  line L14 (-27, 45) -> (-27, 40)
  line L15 (-27, 40) -> (-36, 40)
  line L16 (-36, 40) -> (-36, 45)
  line L17 (-36, 45) -> (-45, 45)
  line L18 (-45, 45) -> (-45, 36)
  line L19 (-45, 36) -> (-40, 36)
  line L20 (-40, 36) -> (-40, 27)
  line L21 (-40, 27) -> (-45, 27)
  line L22 (-45, 27) -> (-45, 18)
  line L23 (-45, 18) -> (-40, 18)
  line L24 (-40, 18) -> (-40, 9)
  line L25 (-40, 9) -> (-45, 9)
  line L26 (-45, 9) -> (-45, 0)
  line L27 (-45, 0) -> (-36, 0)
  line L28 (-36, 0) -> (-36, 5)
  line L29 (-36, 5) -> (-27, 5)
  line L30 (-27, 5) -> (-27, 0)
  line L31 (-27, 0) -> (-18, 0)
  line L32 (-18, 0) -> (-18, 5)
  line L33 (-18, 5) -> (-9, 5)
  line L34 (-9, 5) -> (-9, 0)
  line L35 (-9, 0) -> (0, 0)
  line L36 (-22.5, 0) -> (-22.5, 22.5) construction
  circle A0 centre (-22.5, 22.5) radius 6.5
  dimension "d22" = 22.5
  dimension "d23" = 13
  constraint midpoint L31 L36.start
  constraint perpendicular L13 L36
  constraint coincident L36.end A0.centre
  measures "d22" distance of L36.start L36.end
  measures "d23" diameter of A0
extrude "Extrude2" cut sketch "Sketch2" against normal blind 6 contours A0
sketch "Sketch3" plane through (0, 0, 5) normal (0, 0, 1) x (-1, 0, 0)
  circle A0 centre (-22.5, 22.5) radius 6.5
  line L0 (0, 0) -> (0, 9)
  line L1 (0, 9) -> (-5, 9)
  line L2 (-5, 9) -> (-5, 18)
  line L3 (-5, 18) -> (0, 18)
  line L4 (0, 18) -> (0, 27)
  line L5 (0, 27) -> (-5, 27)
  line L6 (-5, 27) -> (-5, 36)
  line L7 (-5, 36) -> (0, 36)
  line L8 (0, 36) -> (0, 45)
  line L9 (0, 45) -> (-9, 45)
  line L10 (-9, 45) -> (-9, 40)
  line L11 (-9, 40) -> (-18, 40)
  line L12 (-18, 40) -> (-18, 45)
  line L13 (-18, 45) -> (-27, 45)
  line L14 (-27, 45) -> (-27, 40)
  line L15 (-27, 40) -> (-36, 40)
  line L16 (-36, 40) -> (-36, 45)
  line L17 (-36, 45) -> (-45, 45)
  line L18 (-45, 45) -> (-45, 36)
  line L19 (-45, 36) -> (-40, 36)
  line L20 (-40, 36) -> (-40, 27)
  line L21 (-40, 27) -> (-45, 27)
  line L22 (-45, 27) -> (-45, 18)
  line L23 (-45, 18) -> (-40, 18)
  line L24 (-40, 18) -> (-40, 9)
  line L25 (-40, 9) -> (-45, 9)
  line L26 (-45, 9) -> (-45, 0)
  line L27 (-45, 0) -> (-36, 0)
  line L28 (-36, 0) -> (-36, 5)
  line L29 (-36, 5) -> (-27, 5)
  line L30 (-27, 5) -> (-27, 0)
  line L31 (-27, 0) -> (-18, 0)
  line L32 (-18, 0) -> (-18, 5)
  line L33 (-18, 5) -> (-9, 5)
  line L34 (-9, 5) -> (-9, 0)
  line L35 (-9, 0) -> (0, 0)
  line L36 (-28, 12) -> (-38, 12) construction
  line L37 (-38, 12) -> (-38, 8) construction
  line L38 (-38, 8) -> (-28, 8) construction
  line L39 (-28, 8) -> (-28, 12) construction
  dimension "d26" = 3
  text T0 "1001" font "Arial" height 3 align left top in box 10 x 4 at (-28, 12) x (-1, 0) y (0, -1) spacing 1 kerned
emboss "Emboss1" depth -0.1 profiles "Sketch3" section 1 text T0 onto face at (9.2451, -29.9737, 5)

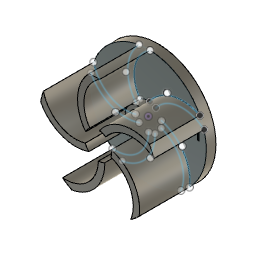
design "Impeller redesigned"
Autodesk Fusion 360 part; units mm, degrees
sketch "Sketch1" plane through (0, 0, 0) normal (0, 1, 0) x (1, 0, 0)
  circle A0 centre (0, 0) radius 15
  line L0 (0, 0) -> (0, 1.5) construction
  line L1 (0, 1.5) -> (2, 1.5)
  line L2 (0, 1.5) -> (-2, 1.5)
  arc A1 (-2, 1.5) -> (2, 1.5) centre (0, 0) ccw
  dimension "d2" = 30
  dimension "d3" = 5
  dimension "d4" = 1.5
  constraint coincident A0.centre L0.start
  constraint concentric A0 A1
  constraint vertical L0
  constraint perpendicular L0 L1
  constraint perpendicular L0 L2
  measures "d2" diameter of A0
  measures "d3" diameter of A1
  measures "d4" distance of A0.centre L0.end
extrude "Extrude1" add sketch "Sketch1" along normal blind 2.5
sketch "Sketch2" plane through (0, 0, 0) normal (0, -1, 0) x (1, 0, 0)
  line L0 (2, -1.5) -> (-2, -1.5)
  arc A0 (2, -1.5) -> (-2, -1.5) centre (0, 0) ccw
  circle A1 centre (0, 0) radius 15
  circle A2 centre (0, 0) radius 3.5
  dimension "d7" = 7
  constraint concentric A0 A2
  measures "d7" diameter of A2
extrude "Extrude2" add sketch "Sketch2" along normal blind 2.5 contours A2
sketch "Sketch3" plane through (0, 0, 0) normal (0, -1, 0) x (1, 0, 0)
  circle A0 centre (0, 0) radius 3.5
  circle A1 centre (0, 0) radius 15
  arc A2 (14.4004, 4.1986) -> (1.9867, 2.8815) centre (8.8128, -2.296) ccw
  arc A3 (13.3375, 6.8638) -> (0.385, 3.4788) centre (8.8128, -2.296) ccw
  arc A4 (0.4568, 14.993) -> (-2.1266, 2.7799) centre (4.9069, 7.6719) ccw
  arc A5 (-2.4063, 14.8057) -> (-3.1895, 1.4412) centre (4.9069, 7.6719) ccw
  arc A6 (-14.1181, 5.0676) -> (-3.301, -1.1634) centre (-5.7801, 7.0375) ccw
  arc A7 (-14.8247, 2.2867) -> (-2.3563, -2.5881) centre (-5.7801, 7.0375) ccw
  arc A8 (-9.1823, -11.8611) -> (0.0864, -3.4989) centre (-8.4792, -3.3225) ccw
  arc A9 (-6.7558, -13.3925) -> (1.7333, -3.0407) centre (-8.4792, -3.3225) ccw
  arc A10 (8.4431, -12.3982) -> (3.3544, -0.999) centre (0.5396, -9.0909) ccw
  arc A11 (10.6493, -10.5637) -> (3.4275, 0.7088) centre (0.5396, -9.0909) ccw
  dimension "d12" = 360
  constraint coincident A1 A2.start
  constraint coincident A0 A2.end
  constraint concentric A2 A3
  constraint coincident A1 A3.start
  constraint coincident A0 A3.end
extrude "Extrude3" add sketch "Sketch3" along normal blind 13 contours A0 A1 A10 A11 | A0 A1 A2 A3 | A0 A1 A8 A9 | A0 A1 A4 A5 | A0 A1 A6 A7
sketch "Sketch4" plane through (0, 0, 0) normal (0, 1, 0) x (1, 0, 0)
  line L0 (5, -1.4452) -> (12.6435, -1.4452) construction
  line L1 (12.6435, -1.4452) -> (12.6435, -4) construction
  line L2 (12.6435, -4) -> (5, -4) construction
  line L3 (5, -4) -> (5, -1.4452) construction
  dimension "d15" = 3
  text T0 "1001" font "Arial" height 3 align left top in box 7.6435 x 2.5548 at (5, -1.4452) x (1, 0) y (0, -1) spacing 1 kerned
emboss "Emboss1" depth -0.2 profiles "Sketch4" section 1 text T0 onto face at (11.4096, 0, 2.3302)
